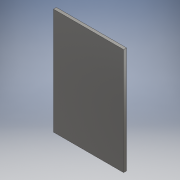
# Autodesk Inventor part: Multi-Inno_3.5in_LCD
Saved by Autodesk Inventor 2017 (Build 210142000, 142)
## iProperties
Created: 2018-08-14
Part Number: Multi-Inno_3.5in_LCD
Material: Generic
Document SubType Name: Modeling
Designer: intelsath
Density: 1 g/cm^3
Appearance: Default
Author: intelsath
Autodesk Inventor part; units mm, degrees
ref_plane "YZ Plane" through (0, 0, 0) normal (1, 0, 0) x (0, 1, 0)
ref_plane "XZ Plane" through (0, 0, 0) normal (0, 1, 0) x (-1, 0, 0)
ref_plane "XY Plane" through (0, 0, 0) normal (0, 0, 1) x (1, 0, 0)
sketch "Sketch1" plane through (0, 0, 0) normal (0, 1, 0) x (-1, 0, 0)
  line L0 (27.33, 41.47) -> (-27.33, 41.47)
  line L1 (-27.33, 41.47) -> (-27.33, -41.47)
  line L2 (-27.33, -41.47) -> (27.33, -41.47)
  line L3 (27.33, -41.47) -> (27.33, 41.47)
  line L4 (27.33, 41.47) -> (-27.33, -41.47) construction
  line L5 (-27.33, 41.47) -> (27.33, -41.47) construction
  point P0 (0, 0)
  dimension "d0" = 82.94
  dimension "d1" = 54.66
  constraints: 12 end point, 2 midpoint, 2 parallel, 1 horizontal, 1 perpendicular
  measures "d0" distance of L0.end L1.end
  measures "d1" distance of L1.end L2.end
extrude "Extrusion1" add sketch "Sketch1" along normal blind 2.3
sketch "Sketch2" plane through (0, 2.3, 0) normal (0, 1, 0) x (1, 0, 0)
  line L0 (-24.98, 39.62) -> (24.98, 39.62)
  line L1 (24.98, 39.62) -> (24.98, -34.82)
  line L2 (24.98, -34.82) -> (-24.98, -34.82)
  line L3 (-24.98, -34.82) -> (-24.98, 39.62)
  line L4 (-24.98, 39.62) -> (24.98, -34.82) construction
  line L5 (24.98, 39.62) -> (-24.98, -34.82) construction
  line L6 (27.33, 41.47) -> (-27.33, 41.47) projected
  point P0 (0, 0)
  point P1 (0, 2.4)
  dimension "d4" = 74.44
  dimension "d5" = 49.96
  dimension "d6" = 1.85
  constraints: 12 end point, 2 midpoint, 2 parallel, 1 horizontal, 1 perpendicular, 1 vertical alignment
  measures "d4" distance of L2.end L0.start
  measures "d5" distance of L1.end L2.end
  measures "d6" distance between parallel lines of L0 L6
extrude "Extrusion2" cut sketch "Sketch2" against normal blind 0.05
body "Solid1"
